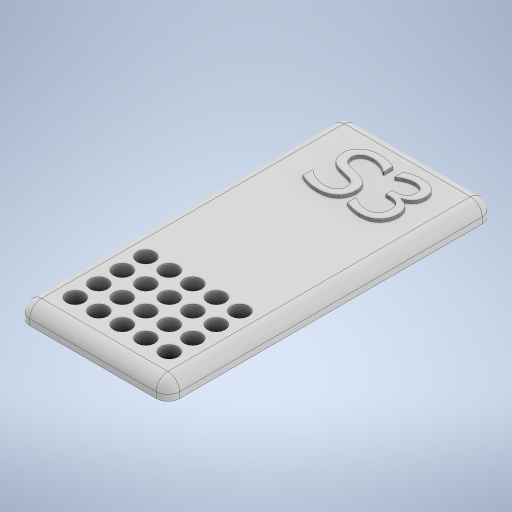
# Autodesk Inventor part: sensor3
Saved by Autodesk Inventor 2024 (Build 280153000, 153)
## iProperties
Created: 2024-03-11
Part Number: sensor3
Material: Generic
Document SubType Name: Modeling
Designer: quinten
Density: 1 g/cm^3
Appearance: Default
Author: quinten
Autodesk Inventor part; units mm, degrees
ref_plane "YZ Plane" through (0, 0, 0) normal (1, 0, 0) x (0, 1, 0)
ref_plane "XZ Plane" through (0, 0, 0) normal (0, 1, 0) x (-1, 0, 0)
ref_plane "XY Plane" through (0, 0, 0) normal (0, 0, 1) x (1, 0, 0)
sketch "Sketch1" plane through (0, 0, 0) normal (0, 1, 0) x (-1, 0, 0)
  line L0 (0, 0) -> (21.5, 0)
  line L1 (21.5, 0) -> (21.5, -51.5)
  line L2 (21.5, -51.5) -> (0, -51.5)
  line L3 (0, -51.5) -> (0, 0)
  line L4 (23.5, 2) -> (-2, 2)
  line L5 (-2, 2) -> (-2, -53.5)
  line L6 (-2, -53.5) -> (23.5, -53.5)
  line L7 (23.5, -53.5) -> (23.5, 2)
  line L8 (10.75, 0) -> (10.75, -51.5) construction
  circle A0 centre (10.75, -3) radius 1.5
  line L9 (0, -3) -> (21.5, -3) construction
  circle A1 centre (14.75, -3) radius 1.5
  circle A2 centre (18.75, -3) radius 1.5
  circle A3 centre (6.75, -3) radius 1.5
  circle A4 centre (2.75, -3) radius 1.5
  circle A5 centre (18.75, -7) radius 1.5
  circle A6 centre (14.75, -7) radius 1.5
  circle A7 centre (10.75, -7) radius 1.5
  circle A8 centre (6.75, -7) radius 1.5
  circle A9 centre (2.75, -7) radius 1.5
  circle A10 centre (18.75, -11) radius 1.5
  circle A11 centre (14.75, -11) radius 1.5
  circle A12 centre (10.75, -11) radius 1.5
  circle A13 centre (6.75, -11) radius 1.5
  circle A14 centre (2.75, -11) radius 1.5
  circle A15 centre (18.75, -15) radius 1.5
  circle A16 centre (14.75, -15) radius 1.5
  circle A17 centre (10.75, -15) radius 1.5
  circle A18 centre (6.75, -15) radius 1.5
  circle A19 centre (2.75, -15) radius 1.5
  point P0 (10.75, -3)
  point P1 (10.75, -7)
  point P2 (10.75, -11)
  point P3 (10.75, -15)
  dimension "d0" = 21.5
  dimension "d1" = 51.5
  dimension "d2" = 2
  dimension "d3" = 2
  dimension "d4" = 2
  dimension "d5" = 2
  dimension "d6" = 3
  dimension "d8" = 3
  dimension "d9" = 3
  dimension "d10" = 3
  dimension "d11" = 3
  dimension "d12" = 3
  dimension "d13" = 4
  dimension "d14" = 4
  dimension "d15" = 4
  dimension "d16" = 4
  dimension "d19" = 4
  constraints: 20 centre point, 20 end point, 7 point on line, 4 midpoint, 4 parallel, 3 perpendicular, 2 horizontal, 1 vertical, 33 other
  measures "d0" distance of L1.end L2.end
  measures "d1" distance of L0.end L1.end
  measures "d2" distance between parallel lines of L7 L1
  measures "d3" distance between parallel lines of L0 L4
  measures "d4" distance between parallel lines of L3 L5
  measures "d5" distance between parallel lines of L6 L2
  measures "d6" diameter of A0
  measures "d8" distance between parallel lines of L0 L9
  measures "d9" diameter of A1
  measures "d10" diameter of A2
  measures "d11" diameter of A3
  measures "d12" diameter of A4
  measures "d13" distance of point (10.75, -3) A3.centre
  measures "d14" distance of A3.centre A4.centre
  measures "d15" distance of A1.centre point (10.75, -3)
  measures "d16" distance of A2.centre A1.centre
  measures "d19" distance of A2.centre A5.centre
extrude "Extrusion1" add sketch "Sketch1" along normal blind 3 contours L0 L1 L2 L3 | L7 L6 L5 L4
fillet "Fillet1" radius 2 8 edges at (-23.5, 3, -25.75) (-10.75, 3, 2) (-23.5, 1.5, 2) (2, 1.5, 2) (2, 3, -25.75) (-10.75, 3, -53.5) (-23.5, 1.5, -53.5) (2, 1.5, -53.5)
sketch "Sketch2" plane through (0, 3, 0) normal (0, 1, 0) x (1, 0, 0)
  line L0 (-17.4247, 49.4836) -> (-8.1758, 49.4836) construction
  line L1 (-8.1758, 49.4836) -> (-8.1758, 43.1661) construction
  line L2 (-8.1758, 43.1661) -> (-17.4247, 43.1661) construction
  line L3 (-17.4247, 43.1661) -> (-17.4247, 49.4836) construction
  spline S0 degree 2 poles (-13.624, 39.0946) (-14.7099, 39.0946) (-16.2334, 39.5484) (-16.906, 39.8726) knots 0 0 0 1 2 2 2
  line L4 (-16.906, 39.8726) -> (-16.906, 41.5419)
  line L5 (-16.906, 41.5419) -> (-16.8088, 41.5419)
  spline S1 degree 2 poles (-16.8088, 41.5419) (-16.1524, 40.9261) (-14.4911, 40.2453) (-13.7213, 40.2453) knots 0 0 0 1 2 2 2
  spline S2 degree 2 poles (-13.7213, 40.2453) (-12.6192, 40.2453) (-11.4928, 41.1611) (-11.4928, 41.9147) knots 0 0 0 1 2 2 2
  spline S3 degree 2 poles (-11.4928, 41.9147) (-11.4928, 42.5144) (-12.0843, 43.2599) (-12.7245, 43.4463) knots 0 0 0 1 2 2 2
  spline S4 degree 2 poles (-12.7245, 43.4463) (-13.1864, 43.576) (-13.9563, 43.7543) (-14.5317, 43.9001) knots 0 0 0 1 2 2 2
  spline S5 degree 2 poles (-14.5317, 43.9001) (-15.0503, 44.0379) (-15.8688, 44.4512) (-16.1848, 44.7834) knots 0 0 0 1 2 2 2
  spline S6 degree 2 poles (-16.1848, 44.7834) (-16.4928, 45.1157) (-16.8331, 46.0071) (-16.8331, 46.5906) knots 0 0 0 1 2 2 2
  spline S7 degree 2 poles (-16.8331, 46.5906) (-16.8331, 47.8061) (-14.9368, 49.4512) (-13.4701, 49.4512) knots 0 0 0 1 2 2 2
  spline S8 degree 2 poles (-13.4701, 49.4512) (-12.6273, 49.4512) (-11.1362, 49.1189) (-10.496, 48.8029) knots 0 0 0 1 2 2 2
  line L6 (-10.496, 48.8029) -> (-10.496, 47.2146)
  line L7 (-10.496, 47.2146) -> (-10.5932, 47.2146)
  spline S9 degree 2 poles (-10.5932, 47.2146) (-11.0714, 47.6522) (-12.5624, 48.3005) (-13.3809, 48.3005) knots 0 0 0 1 2 2 2
  spline S10 degree 2 poles (-13.3809, 48.3005) (-14.3047, 48.3005) (-15.4474, 47.4334) (-15.4474, 46.7283) knots 0 0 0 1 2 2 2
  spline S11 degree 2 poles (-15.4474, 46.7283) (-15.4474, 46.0962) (-14.7748, 45.3426) (-14.1427, 45.1724) knots 0 0 0 1 2 2 2
  spline S12 degree 2 poles (-14.1427, 45.1724) (-13.7213, 45.059) (-12.4976, 44.7672) (-12.0924, 44.6457) knots 0 0 0 1 2 2 2
  spline S13 degree 2 poles (-12.0924, 44.6457) (-11.0633, 44.3296) (-10.107, 43.0573) (-10.107, 42.1254) knots 0 0 0 1 2 2 2
  spline S14 degree 2 poles (-10.107, 42.1254) (-10.107, 41.5338) (-10.5851, 40.3993) (-11.0146, 40.0022) knots 0 0 0 1 2 2 2
  spline S15 degree 2 poles (-11.0146, 40.0022) (-11.4928, 39.5646) (-12.7083, 39.0946) (-13.624, 39.0946) knots 0 0 0 1 2 2 2
  spline S16 degree 2 poles (-6.3388, 48.3248) (-6.7035, 48.3248) (-7.4247, 48.1465) (-7.7731, 48.0087) knots 0 0 0 1 2 2 2
  spline S17 degree 2 poles (-7.7731, 48.0087) (-8.0973, 47.871) (-8.5754, 47.5792) (-8.7618, 47.4496) knots 0 0 0 1 2 2 2
  line L8 (-8.7618, 47.4496) -> (-8.8428, 47.4496)
  line L9 (-8.8428, 47.4496) -> (-8.8428, 48.8677)
  spline S18 degree 2 poles (-8.8428, 48.8677) (-8.4052, 49.1027) (-6.906, 49.4836) (-6.2334, 49.4836) knots 0 0 0 1 2 2 2
  spline S19 degree 2 poles (-6.2334, 49.4836) (-5.5527, 49.4836) (-4.5398, 49.2081) (-4.1265, 48.9163) knots 0 0 0 1 2 2 2
  spline S20 degree 2 poles (-4.1265, 48.9163) (-3.6889, 48.6003) (-3.2351, 47.6846) (-3.2351, 47.0687) knots 0 0 0 1 2 2 2
  spline S21 degree 2 poles (-3.2351, 47.0687) (-3.2351, 46.2421) (-4.321, 44.9941) (-5.0827, 44.8321) knots 0 0 0 1 2 2 2
  line L10 (-5.0827, 44.8321) -> (-5.0827, 44.7348)
  spline S22 degree 2 poles (-5.0827, 44.7348) (-4.7667, 44.67) (-4.0454, 44.3782) (-3.7375, 44.0865) knots 0 0 0 1 2 2 2
  spline S23 degree 2 poles (-3.7375, 44.0865) (-3.4295, 43.8029) (-3.0406, 42.8953) (-3.0406, 42.2389) knots 0 0 0 1 2 2 2
  spline S24 degree 2 poles (-3.0406, 42.2389) (-3.0406, 41.5663) (-3.5025, 40.4236) (-3.9239, 39.986) knots 0 0 0 1 2 2 2
  spline S25 degree 2 poles (-3.9239, 39.986) (-4.3615, 39.5322) (-5.6013, 39.0622) (-6.3874, 39.0622) knots 0 0 0 1 2 2 2
  spline S26 degree 2 poles (-6.3874, 39.0622) (-7.1411, 39.0622) (-8.6159, 39.4269) (-9.1184, 39.6781) knots 0 0 0 1 2 2 2
  line L11 (-9.1184, 39.6781) -> (-9.1184, 41.0962)
  line L12 (-9.1184, 41.0962) -> (-9.0211, 41.0962)
  spline S27 degree 2 poles (-9.0211, 41.0962) (-8.5997, 40.7883) (-7.1735, 40.221) (-6.4684, 40.221) knots 0 0 0 1 2 2 2
  spline S28 degree 2 poles (-6.4684, 40.221) (-6.0552, 40.221) (-5.2286, 40.4804) (-4.953, 40.7802) knots 0 0 0 1 2 2 2
  spline S29 degree 2 poles (-4.953, 40.7802) (-4.6856, 41.08) (-4.402, 41.7932) (-4.402, 42.3361) knots 0 0 0 1 2 2 2
  spline S30 degree 2 poles (-4.402, 42.3361) (-4.402, 42.8791) (-4.718, 43.5841) (-5.0017, 43.7867) knots 0 0 0 1 2 2 2
  spline S31 degree 2 poles (-5.0017, 43.7867) (-5.2853, 43.9893) (-6.0552, 44.1432) (-6.509, 44.1432) knots 0 0 0 1 2 2 2
  line L13 (-6.509, 44.1432) -> (-7.0762, 44.1432)
  line L14 (-7.0762, 44.1432) -> (-7.0762, 45.2534)
  line L15 (-7.0762, 45.2534) -> (-6.6305, 45.2534)
  spline S32 degree 2 poles (-6.6305, 45.2534) (-5.731, 45.2534) (-4.5965, 46.1124) (-4.5965, 46.9309) knots 0 0 0 1 2 2 2
  spline S33 degree 2 poles (-4.5965, 46.9309) (-4.5965, 47.3118) (-4.8882, 47.8547) (-5.1232, 48.0168) knots 0 0 0 1 2 2 2
  spline S34 degree 2 poles (-5.1232, 48.0168) (-5.3744, 48.187) (-5.9903, 48.3248) (-6.3388, 48.3248) knots 0 0 0 1 2 2 2
  point P0 (0, 0)
  constraints: 2 other
extrude "Extrusion2" add sketch "Sketch2" along normal blind 0.5
equation "\"d8\" = d6"
equation "\"d9\" = d11"
equation "\"d10\" = d11"
equation "\"d11\" = d6"
equation "\"d12\" = d11"
equation "\"d14\" = d13"
equation "\"d15\" = d13"
equation "\"d16\" = d15"
body "Solid1"
